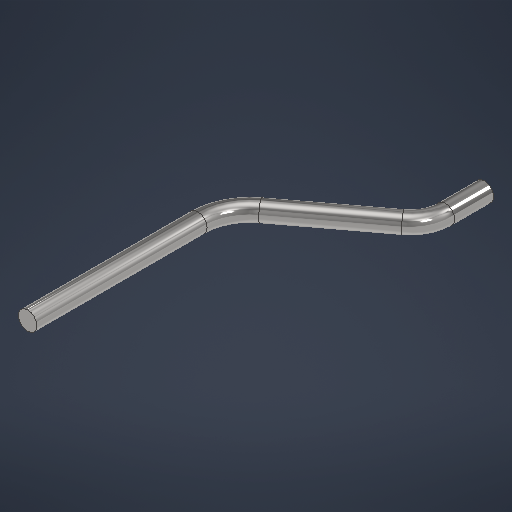
# Autodesk Inventor part: rear iron bar
Saved by Autodesk Inventor 2026.1 (Build 301233000, 233)
## iProperties
Created: 2025-12-10
Part Number: rear iron bar
Material: Generisch
Document SubType Name: Modeling
Designer: Familie
Density: 1 g/cm^3
Appearance: Stahl - poliert
Author: Familie
Autodesk Inventor part; units mm, degrees
ref_plane "YZ Plane" through (0, 0, 0) normal (1, 0, 0) x (0, 1, 0)
ref_plane "XZ Plane" through (0, 0, 0) normal (0, 1, 0) x (-1, 0, 0)
ref_plane "XY Plane" through (0, 0, 0) normal (0, 0, 1) x (1, 0, 0)
sketch "Skizze1" plane through (0, 0, 0) normal (0, 0, 1) x (1, 0, 0)
  line L0 (0, 0) -> (0, 30)
  arc A0 (4.5, 39) -> (0, 30) centre (11.25, 30) ccw
  line L1 (4.5, 39) -> (22, 52.125)
  arc A1 (22, 52.125) -> (25, 58.125) centre (17.5, 58.125) ccw
  line L2 (25, 58.125) -> (25, 60)
  line L3 (25, 60) -> (25, 66.5)
  line L4 (0, 0) -> (0, -6.5)
  dimension "d4" = 30
  dimension "d5" = 60
  dimension "d6" = 25
  dimension "d16" = 4.5
  dimension "d17" = 9
  dimension "d18" = 3
  dimension "d19" = 6.5
  dimension "d20" = 6.5
  constraints: 10 end point, 4 point on circle, 4 tangent, 4 vertical, 2 centre point
  measures "d4" distance of L0.start L0.end
  measures "d5" vertical distance of L0.start L2.end
  measures "d6" horizontal distance of L0.start L2.end
  measures "d16" horizontal distance of L0.end L1.start
  measures "d17" vertical distance of L0.end L1.start
  measures "d18" horizontal distance of L1.end L2.start
  measures "d19" distance of L2.end L3.end
  measures "d20" distance of L0.start L4.end
sketch "Skizze2" plane through (0, 0, 0) normal (0, 1, 0) x (-1, 0, 0)
  circle A0 centre (0, 0) radius 2
  dimension "d1" = 4
  constraints: 1 centre point, 1 coincident
  measures "d1" diameter of A0
sweep "Sweeping1" add profiles "Skizze2" path "Skizze1"
equation "\"d20\" = d19"
